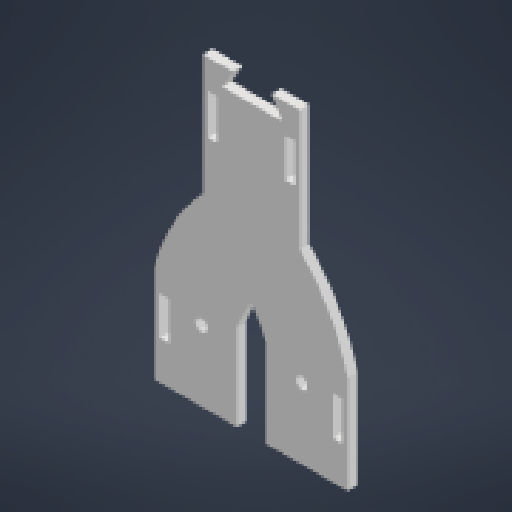
# Autodesk Inventor part: newmiddle
Saved by Autodesk Inventor 2026.2 (Build 302298000, 298)
## iProperties
Created: 2026-04-08
Part Number: newmiddle
Material: Generic
Document SubType Name: Modeling
Designer: danda
Density: 1 g/cm^3
Appearance: Default
Author: danda
Autodesk Inventor part; units mm, degrees
ref_plane "YZ Plane" through (0, 0, 0) normal (1, 0, 0) x (0, 1, 0)
ref_plane "XZ Plane" through (0, 0, 0) normal (0, 1, 0) x (-1, 0, 0)
ref_plane "XY Plane" through (0, 0, 0) normal (0, 0, 1) x (1, 0, 0)
sketch "Sketch1" plane through (0, 0, 0) normal (0, 0, 1) x (1, 0, 0)
  line L0 (48.7872, 31.5555) -> (48.7872, -28.4445)
  line L1 (13.7872, 31.5555) -> (13.7872, -28.4445)
  arc A0 (13.7872, -28.4445) -> (-11.2128, -71.7458) centre (76.1621, -93.3242) ccw
  line L2 (13.7872, -28.4445) -> (-11.2128, -71.7458) construction
  line L3 (13.7872, -28.4445) -> (63.7872, -28.4445) construction
  line L4 (-11.2128, -71.7458) -> (-11.2128, -121.7458)
  arc A1 (73.6491, -71.1938) -> (48.7872, -28.4445) centre (-13.5876, -93.3242) ccw
  line L5 (73.6491, -71.1938) -> (73.6491, -121.1332)
  line L6 (23.7872, -121.7458) -> (23.7872, -76.5352)
  arc A2 (31.2872, -61.5241) -> (23.7872, -76.5352) centre (76.1621, -93.3242) ccw
  arc A3 (38.6491, -76.1101) -> (31.2872, -61.5241) centre (-13.5876, -93.3242) ccw
  line L7 (38.6491, -76.1101) -> (38.6491, -121.1332)
  line L8 (-18.7128, -121.1332) -> (-18.7128, -70.8519)
  arc A4 (6.2872, -25.326) -> (-18.7128, -70.8519) centre (76.1621, -93.3242) ccw
  line L9 (6.2872, -25.326) -> (6.2872, 37.168)
  line L10 (6.2872, 37.168) -> (56.2872, 37.168)
  line L11 (56.2872, 37.168) -> (56.2872, -25.326)
  arc A5 (81.2182, -70.5622) -> (56.2872, -25.326) centre (-13.5876, -93.3242) ccw
  line L12 (81.2182, -70.5622) -> (81.2182, -121.1332)
  line L13 (-18.7128, -121.1332) -> (81.2182, -121.1332)
  line L14 (13.7872, 31.5555) -> (13.7872, 37.168)
  line L15 (48.7872, 31.5555) -> (48.7872, 37.168)
  line L16 (33.6491, -121.1332) -> (33.6491, -85.5895)
  line L17 (28.7872, -85.5895) -> (28.7872, -121.7458)
  line L18 (23.7872, -85.5895) -> (28.7872, -85.5895)
  line L19 (33.6491, -85.5895) -> (38.6491, -85.5895)
  line L20 (48.4283, 31.5555) -> (48.7872, 31.5555)
  line L21 (13.7872, 2.168) -> (13.7872, 22.168)
  line L22 (48.7872, 2.168) -> (48.7872, 22.168)
  line L23 (73.6491, -101.1332) -> (73.6491, -81.1332)
  line L24 (-11.2128, -81.1332) -> (-11.2128, -101.1332)
  line L25 (79.0378, -80.1332) -> (84.0378, -80.1332)
  line L26 (84.0378, -80.1332) -> (84.0378, -101.1332)
  line L27 (48.7872, 1.168) -> (48.7872, 22.168)
  line L28 (8.7872, 22.168) -> (13.7872, 22.168)
  line L29 (13.7872, 22.168) -> (13.7872, 1.168)
  line L30 (13.7872, 1.168) -> (8.7872, 1.168)
  line L31 (8.7872, 1.168) -> (8.7872, 22.168)
  line L32 (48.7872, 22.168) -> (53.7877, 22.168)
  line L33 (53.7877, 22.168) -> (53.7877, 2.168)
  line L34 (53.7877, 2.168) -> (48.7872, 2.168)
  line L35 (48.7872, 2.168) -> (48.7872, 22.168)
  line L36 (21.7872, 37.168) -> (16.2872, 27.6417)
  line L37 (21.7872, 37.168) -> (32.7872, 37.168) construction
  line L38 (16.2872, 27.6417) -> (47.2872, 27.6417)
  line L39 (47.2872, 27.6417) -> (41.7872, 37.168)
  line L40 (-11.2128, -81.1332) -> (-16.2128, -81.1332)
  line L41 (-16.2128, -81.1332) -> (-16.2128, -101.1332)
  line L42 (-16.2128, -101.1332) -> (-11.2128, -101.1332)
  line L43 (-11.2128, -101.1332) -> (-11.2128, -81.1332)
  line L44 (73.6491, -81.1332) -> (78.6491, -81.1332)
  line L45 (78.6491, -81.1332) -> (78.6491, -101.1332)
  line L46 (78.6491, -101.1332) -> (73.6491, -101.1332)
  line L47 (73.6491, -101.1332) -> (73.6491, -81.1332)
  point P0 (0, 0)
  point P1 (-11.2128, -121.1332)
  point P2 (23.7872, -121.1332)
  point P3 (36.2872, -121.7458)
  point P4 (71.2872, -121.7458)
  point P5 (28.7872, -121.1332)
  point P6 (31.2872, -121.7458)
  point P7 (81.2182, -80.1332)
  point P8 (13.7872, 22.168)
  point P9 (13.7872, 1.168)
  point P10 (48.7872, 2.168)
  point P11 (48.7872, 22.168)
  dimension "d0" = 35
  dimension "d1" = 60
  dimension "d2" = 50
  dimension "d3" = 120
  dimension "d4" = 90
  dimension "d5" = 50
  dimension "d6" = 35
  dimension "d7" = 7.5
  dimension "d12" = 5
  dimension "d16" = 7.5
  dimension "d22" = 158.3013
  dimension "d29" = 0
  dimension "d31" = 21
  dimension "d36" = 5
  dimension "d37" = 21
  dimension "d39" = 15
  dimension "d44" = 2.5
  dimension "d45" = 15
  dimension "d46" = 5.0004
  dimension "d47" = 20
  dimension "d48" = 90
  dimension "d49" = 90
  dimension "d50" = 2.8196
  dimension "d51" = 10.3887
  dimension "d52" = 27.7505
  dimension "d53" = 30.2501
  dimension "d54" = 45.3887
  dimension "d55" = 55.2505
  dimension "d58" = 111.6887
  dimension "d59" = 51.6887
  dimension "d60" = 5.4563
  dimension "d61" = 84.0378
  dimension "d62" = 80.1333
  dimension "d63" = 9.571
  dimension "d64" = 1
  dimension "d66" = 12.7505
  dimension "d67" = 41.6125
  dimension "d68" = 102.3013
  dimension "d69" = 82.3013
  dimension "d70" = 81.3013
  dimension "d71" = 47.7505
  dimension "d72" = 41.6125
  dimension "d73" = 52.7505
  dimension "d74" = 41.6125
  dimension "d75" = 55.2505
  dimension "d76" = 41
  dimension "d77" = 41.6125
  dimension "d78" = 60.2505
  dimension "d79" = 41
  dimension "d80" = 41.6125
  dimension "d81" = 102.3013
  dimension "d82" = 82.3013
  dimension "d83" = 1
  dimension "d84" = 21
  dimension "d85" = 95.2505
  dimension "d86" = 41
  dimension "d87" = 11
  dimension "d88" = 120
  dimension "d89" = 31
  dimension "d90" = 11
  dimension "d91" = 60
  dimension "d92" = 14.5
  dimension "d93" = 5
  dimension "d94" = 20
  constraints: 96 end point, 15 point on line, 14 parallel, 12 point on circle, 10 horizontal, 10 perpendicular, 6 centre point, 2 equal length, 2 vertical, 1 equal radius, 5 other
  measures "d0" distance of L1.start L0.start
  measures "d1" distance of L0.start L0.end
  measures "d2" distance of L1.end L2.end
  measures "d3" angle of L2 L3
  measures "d4" radius of A0
  measures "d5" distance of L2.end L4.end
  measures "d6" distance between parallel lines of L4 L6
  measures "d7" distance between parallel lines of L1 L9
  measures "d12" distance between parallel lines of L7 L16
  measures "d16" distance between parallel lines of L11 L0
  measures "d22" distance between parallel lines of L13 L10
  measures "d29" distance between parallel lines of L4 L24
  measures "d31" distance of L25.end L26.end
  measures "d36" distance of L29.end L30.end
  measures "d37" distance of L28.end L29.end
  measures "d39" distance between parallel lines of L10 L28
  measures "d44" distance between parallel lines of L9 L31
  measures "d45" distance between parallel lines of L10 L32
  measures "d46" distance of L33.end L34.end
  measures "d47" distance of L32.end L33.end
  measures "d48" angle of L25 L5
  measures "d49" angle of L27 L25
  measures "d50" distance between parallel lines of L12 L26
  measures "d51" distance between parallel lines of L23 L26
  measures "d52" distance between parallel lines of L26 L11
  measures "d53" distance between parallel lines of L26 L33
  measures "d54" distance between parallel lines of L26 L7
  measures "d55" distance between parallel lines of L17 L26
  measures "d58" distance between parallel lines of L25 L20
  measures "d59" distance between parallel lines of L25 L3
  measures "d60" distance between parallel lines of L25 L18
  measures "d61" distance from line of point (0, 0) L26
  measures "d62" distance from line of point (0, 0) L25
  measures "d63" distance from line of L12.start L25
  measures "d64" distance from line of L23.end L25
  measures "d66" distance from line of point (71.287, -121.746) L26
  measures "d67" distance from line of point (71.287, -121.746) L25
  measures "d68" distance from line of L22.end L25
  measures "d69" distance from line of L22.start L25
  measures "d70" distance from line of L27.start L25
  measures "d71" distance from line of point (36.287, -121.746) L26
  measures "d72" distance from line of point (36.287, -121.746) L25
  measures "d73" distance from line of point (31.287, -121.746) L26
  measures "d74" distance from line of point (31.287, -121.746) L25
  measures "d75" distance from line of point (28.787, -121.133) L26
  measures "d76" distance from line of point (28.787, -121.133) L25
  measures "d77" distance from line of L17.end L25
  measures "d78" distance from line of point (23.787, -121.133) L26
  measures "d79" distance from line of point (23.787, -121.133) L25
  measures "d80" distance from line of L6.start L25
  measures "d81" distance from line of L21.end L25
  measures "d82" distance from line of L21.start L25
  measures "d83" distance from line of L24.start L25
  measures "d84" distance from line of L24.end L25
  measures "d85" distance from line of point (-11.213, -121.133) L26
  measures "d86" distance from line of point (-11.213, -121.133) L25
  measures "d87" distance of L37.start L36.end
  measures "d88" angle of L36 L37
  measures "d89" distance of L36.end L39.start
  measures "d90" distance of L39.start L39.end
  measures "d91" angle of L38 L39
  measures "d92" distance of L10.end L39.end
  measures "d93" distance of L42.end L41.end
  measures "d94" distance of L41.end L40.end
extrude "Extrusion1" add sketch "Sketch1" along normal blind 5 contours L15 L10 L11 A5 L12 L13 L5 L46 L45 L44 A1 L0 L34 L33 L32 | L0 A1 L5 L13 L7 A3 A2 L6 L4 A0 L1 L14 L10 L36 L38 L39 L15 | L14 L1 L28 L31 L30 A0 L4 L40 L41 L42 L13 L8 A4 L9 L10
sketch "Sketch2" plane through (0, 0, 5) normal (0, 0, 1) x (1, 0, 0)
  circle A0 centre (57.4252, -84.5438) radius 3
  circle A1 centre (5.4252, -84.5438) radius 3
  point P0 (0, 0)
  dimension "d99" = 6
  dimension "d100" = 6
  dimension "d101" = 52
  constraints: 2 centre point
  measures "d99" diameter of A0
  measures "d100" diameter of A1
  measures "d101" distance of A0.centre A1.centre
extrude "Extrusion3" cut sketch "Sketch2" against normal blind 5
equation "\"d16\" = d7"
body "Solid1"
